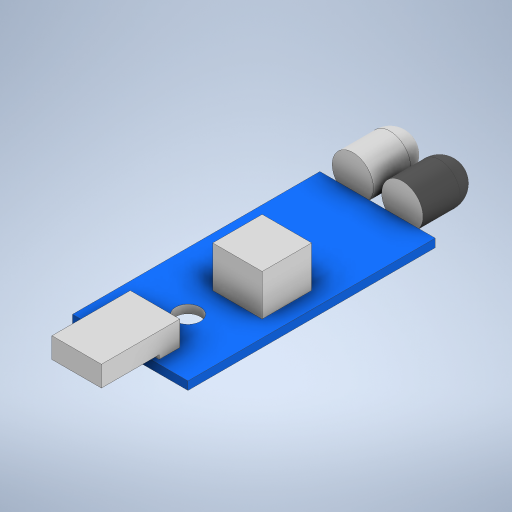
# Autodesk Inventor part: IR
Saved by Autodesk Inventor 2024.2 (Build 282272000, 272)
## iProperties
Created: 2024-05-04
Part Number: IR
Material: Generic
Document SubType Name: Modeling
Designer: ringl
Density: 1 g/cm^3
Appearance: Default
Author: ringl
Autodesk Inventor part; units mm, degrees
ref_plane "YZ Plane" through (0, 0, 0) normal (1, 0, 0) x (0, 1, 0)
ref_plane "XZ Plane" through (0, 0, 0) normal (0, 1, 0) x (-1, 0, 0)
ref_plane "XY Plane" through (0, 0, 0) normal (0, 0, 1) x (1, 0, 0)
sketch "Sketch1" plane through (0, 0, 0) normal (0, 1, 0) x (-1, 0, 0)
  line L0 (0, 0) -> (14, 0)
  line L1 (14, 0) -> (14, -30)
  line L2 (14, -30) -> (0, -30)
  line L3 (0, -30) -> (0, 0)
  dimension "d0" = 14
  dimension "d1" = 30
  constraints: 8 end point, 2 parallel, 1 horizontal, 1 perpendicular
  measures "d0" distance of L1.end L2.end
  measures "d1" distance of L0.end L1.end
extrude "Extrusion1" add sketch "Sketch1" along normal blind 1
sketch "Sketch2" plane through (0, 0, -30) normal (0, 0, -1) x (-1, 0, 0)
  circle A0 centre (4, 2.5) radius 2.5
  circle A1 centre (10, 2.5) radius 2.5
  line L0 (0, 0) -> (14, 0) projected
  line L1 (14, 0) -> (14, 1) projected
  line L2 (0, 0) -> (0, 1) projected
  point P0 (14, 0.5)
  point P1 (0, 0.5)
  dimension "d4" = 5
  dimension "d5" = 5
  dimension "d6" = 2.5
  dimension "d7" = 4
  dimension "d8" = 4
  constraints: 2 centre point, 2 midpoint, 1 horizontal alignment
  measures "d4" diameter of A0
  measures "d5" diameter of A1
  measures "d6" distance from line of A1.centre L0
  measures "d7" horizontal distance of point (14, 0.5) A1.centre
  measures "d8" horizontal distance of point (0, 0.5) A0.centre
extrude "Extrusion2" add sketch "Sketch2" along normal blind 7
fillet "Fillet1" radius 2.5 2 edges at (-1.5, 2.5, -37) (-7.5, 2.5, -37)
sketch "Sketch3" plane through (0, 1, 0) normal (0, 1, 0) x (1, 0, 0)
  line L0 (-10, 0.5) -> (-4, 0.5)
  line L1 (-4, 0.5) -> (-4, 3)
  line L2 (-4, 3) -> (-10, 3)
  line L3 (-10, 3) -> (-10, 0.5)
  line L4 (0, 0) -> (0, 30) projected
  line L5 (-14, 0) -> (0, 0) projected
  point P0 (-7, 0.5)
  dimension "d12" = 6
  dimension "d13" = 4
  dimension "d14" = 2.5
  dimension "d15" = 0.5
  constraints: 8 end point, 2 parallel, 1 horizontal, 1 midpoint, 1 perpendicular
  measures "d12" distance of L2.end L1.end
  measures "d13" distance between parallel lines of L4 L1
  measures "d14" distance between parallel lines of L0 L2
  measures "d15" distance from line of L5 point (-7, 0.5)
extrude "Extrusion3" add sketch "Sketch3" along normal blind 3
sketch "Sketch4" plane through (-10, 1, -0.5) normal (0, 0, 1) x (1, 0, 0)
  line L0 (6, 3) -> (0, 3) projected
  line L1 (6, 0) -> (6, 3) projected
  line L2 (0, 3) -> (6, 3)
  line L3 (6, 3) -> (6, 0.5)
  line L4 (6, 0.5) -> (0, 0.5)
  line L5 (0, 0.5) -> (0, 3)
  point P0 (10, -1)
  dimension "d18" = 2.5
  constraints: 8 end point, 2 parallel, 1 horizontal, 1 perpendicular, 1 point on line
  measures "d18" distance between parallel lines of L0 L4
extrude "Extrusion4" add sketch "Sketch4" along normal blind 7
sketch "Sketch5" plane through (0, 1, 0) normal (0, 1, 0) x (1, 0, 0)
  line L0 (-2, 17) -> (-8, 17)
  line L1 (-8, 17) -> (-8, 11)
  line L2 (-8, 11) -> (-2, 11)
  line L3 (-2, 11) -> (-2, 17)
  line L4 (0, 0) -> (0, 30) projected
  line L5 (-1.5, 30) -> (-6.5, 30) projected
  point P0 (-2, 14)
  point P1 (-6, 30)
  point P2 (-2, 30)
  dimension "d21" = 6
  dimension "d22" = 6
  dimension "d23" = 2
  dimension "d24" = 13
  constraints: 8 end point, 2 parallel, 1 horizontal, 1 midpoint, 1 perpendicular
  measures "d21" distance of L2.end L1.end
  measures "d22" distance of L1.end L0.end
  measures "d23" distance from line of L4 point (-2, 14)
  measures "d24" distance between parallel lines of L5 L0
extrude "Extrusion5" add sketch "Sketch5" along normal blind 5
sketch "Sketch6" plane through (0, 1, 0) normal (0, 1, 0) x (1, 0, 0)
  circle A0 centre (-7, 7) radius 1.5
  line L0 (-14, 0) -> (0, 0) projected
  line L1 (0, 0) -> (0, 30) projected
  dimension "d27" = 3
  dimension "d28" = 7
  dimension "d29" = 7
  constraints: 1 centre point
  measures "d27" diameter of A0
  measures "d28" distance from line of L0 A0.centre
  measures "d29" distance from line of A0.centre L1
extrude "Extrusion6" cut sketch "Sketch6" against normal through all
body "Solid1"
